Autodesk Fusion 360 part; units mm, degrees
note: some values were not read from the file. Set by a fixed rule: which sketch regions a step uses.
(part 9 of 15)
  line L7029 (253.402, -123.809) -> (253.455, -123.987)
  line L7030 (75.174, -122.125) -> (75.3489, -121.903)
  line L7031 (253.455, -123.987) -> (253.474, -124.171)
  line L7032 (253.45, -124.382) -> (253.391, -124.558)
  line L7033 (252.688, -125.107) -> (252.504, -125.121)
  line L7034 (82.7574, -124.342) -> (82.6989, -124.518)
  line L7035 (82.6989, -124.518) -> (82.6073, -124.679)
  line L7036 (82.34, -124.934) -> (82.1745, -125.017)
  line L7037 (252.53, -123.222) -> (252.715, -123.241)
  line L7038 (82.7806, -124.158) -> (82.7574, -124.342)
  line L7039 (82.6073, -124.679) -> (82.4861, -124.819)
  line L7040 (82.1991, -123.256) -> (82.3622, -123.344)
  line L7041 (82.1745, -125.017) -> (81.996, -125.067)
  line L7042 (81.996, -125.067) -> (81.8111, -125.081)
  line L7043 (82.7093, -123.769) -> (82.7629, -123.947)
  line L7044 (251.981, -124.952) -> (251.84, -124.831)
  line L7045 (251.859, -123.493) -> (252.003, -123.377)
  line L7046 (277.272, -120.321) -> (277.535, -120.423)
  line L7047 (278.68, -122.358) -> (278.642, -122.638)
  line L7048 (82.5051, -123.462) -> (82.6223, -123.606)
  line L7049 (251.74, -123.635) -> (251.859, -123.493)
  line L7050 (276.997, -120.257) -> (277.272, -120.321)
  line L7051 (82.4861, -124.819) -> (82.34, -124.934)
  line L7052 (252.32, -125.099) -> (252.143, -125.042)
  line L7053 (81.8376, -123.181) -> (82.022, -123.201)
  line L7054 (75.5533, -121.708) -> (75.7832, -121.544)
  line L7055 (253.055, -123.384) -> (253.198, -123.502)
  line L7056 (278.566, -122.91) -> (278.451, -123.168)
  line L7057 (278.604, -121.675) -> (278.664, -121.951)
  line L7058 (252.143, -125.042) -> (251.981, -124.952)
  line L7059 (251.64, -124.521) -> (251.589, -124.343)
  line L7060 (81.653, -123.198) -> (81.8376, -123.181)
  line L7061 (81.627, -125.059) -> (81.4507, -125.002)
  line L7062 (81.0324, -124.646) -> (80.9477, -124.481)
  line L7063 (278.007, -120.732) -> (278.205, -120.934)
  line L7064 (251.84, -124.831) -> (251.725, -124.686)
  line L7065 (82.7629, -123.947) -> (82.781, -124.131)
  line L7066 (252.346, -123.238) -> (252.53, -123.222)
  line L7067 (251.589, -124.343) -> (251.574, -124.158)
  line L7068 (278.373, -121.161) -> (278.507, -121.41)
  line L7069 (82.6223, -123.606) -> (82.7093, -123.769)
  line L7070 (251.594, -123.974) -> (251.65, -123.797)
  line L7071 (278.684, -122.233) -> (278.68, -122.358)
  line L7072 (278.642, -122.638) -> (278.566, -122.91)
  line L7073 (252.168, -123.291) -> (252.346, -123.238)
  line L7074 (253.198, -123.502) -> (253.315, -123.646)
  line L7075 (278.451, -123.168) -> (278.302, -123.408)
  line L7076 (82.3622, -123.344) -> (82.5051, -123.462)
  line L7077 (278.205, -120.934) -> (278.373, -121.161)
  line L7078 (80.9477, -124.481) -> (80.8966, -124.303)
  line L7079 (252.003, -123.377) -> (252.168, -123.291)
  line L7080 (76.8596, -121.25) -> (77.141, -121.274)
  line L7081 (278.507, -121.41) -> (278.604, -121.675)
  line L7082 (81.3108, -123.336) -> (81.4751, -123.251)
  line L7083 (277.782, -120.561) -> (278.007, -120.732)
  line L7084 (253.3, -124.719) -> (253.179, -124.859)
  line L7085 (253.315, -123.646) -> (253.402, -123.809)
  line L7086 (81.4751, -123.251) -> (81.653, -123.198)
  line L7087 (81.0471, -123.595) -> (81.1663, -123.453)
  line L7088 (80.9578, -123.757) -> (81.0471, -123.595)
  line L7089 (82.781, -124.131) -> (82.7806, -124.158)
  line L7090 (278.664, -121.951) -> (278.684, -122.233)
  line L7091 (277.535, -120.423) -> (277.782, -120.561)
  line L7092 (82.022, -123.201) -> (82.1991, -123.256)
  line L7093 (251.725, -124.686) -> (251.64, -124.521)
  line L7094 (251.65, -123.797) -> (251.74, -123.635)
  line L7095 (76.3004, -121.32) -> (76.5775, -121.265)
  line L7096 (251.574, -124.158) -> (251.594, -123.974)
  line L7097 (253.179, -124.859) -> (253.033, -124.974)
  line L7098 (57.8588, -124.184) -> (57.5764, -124.19)
  line L7099 (58.1375, -124.137) -> (57.8588, -124.184)
  line L7100 (55.7334, -122.69) -> (55.6827, -122.412)
  line L7101 (58.5222, -120.383) -> (58.7687, -120.521)
  line L7102 (81.1663, -123.453) -> (81.3108, -123.336)
  line L7103 (275.03, -121.108) -> (275.205, -120.887)
  line L7104 (278.12, -123.624) -> (277.91, -123.813)
  line L7105 (277.42, -124.092) -> (277.151, -124.177)
  line L7106 (59.1069, -123.584) -> (58.8964, -123.773)
  line L7107 (275.205, -120.887) -> (275.409, -120.692)
  line L7108 (276.036, -124.125) -> (275.776, -124.015)
  line L7109 (55.8229, -122.958) -> (55.7334, -122.69)
  line L7110 (275.639, -120.527) -> (275.89, -120.397)
  line L7111 (59.5912, -121.635) -> (59.6507, -121.911)
  line L7112 (57.0228, -124.085) -> (56.7626, -123.975)
  line L7113 (58.9932, -120.692) -> (59.1914, -120.894)
  line L7114 (59.5524, -122.87) -> (59.4381, -123.128)
  line L7115 (276.156, -120.304) -> (276.433, -120.248)
  line L7116 (274.836, -122.998) -> (274.747, -122.73)
  line L7117 (58.2587, -120.281) -> (58.5222, -120.383)
  line L7118 (276.433, -120.248) -> (276.715, -120.233)
  line L7119 (276.59, -124.23) -> (276.309, -124.197)
  line L7120 (274.782, -121.615) -> (274.888, -121.353)
  line L7121 (57.9835, -120.217) -> (58.2587, -120.281)
  line L7122 (274.685, -122.17) -> (274.714, -121.889)
  line L7123 (276.309, -124.197) -> (276.036, -124.125)
  line L7124 (278.302, -123.408) -> (278.12, -123.624)
  line L7125 (57.5764, -124.19) -> (57.2959, -124.157)
  line L7126 (81.2888, -124.912) -> (81.1476, -124.791)
  line L7127 (80.9017, -123.934) -> (80.9578, -123.757)
  line L7128 (274.888, -121.353) -> (275.03, -121.108)
  line L7129 (56.5206, -123.829) -> (56.3015, -123.65)
  line L7130 (56.3015, -123.65) -> (56.1098, -123.443)
  line L7131 (59.3593, -121.121) -> (59.4934, -121.37)
  line L7132 (58.7687, -120.521) -> (58.9932, -120.692)
  line L7133 (55.6716, -122.13) -> (55.7004, -121.849)
  line L7134 (276.872, -124.224) -> (276.59, -124.23)
  line L7135 (275.89, -120.397) -> (276.156, -120.304)
  line L7136 (81.4507, -125.002) -> (81.2888, -124.912)
  line L7137 (81.1476, -124.791) -> (81.0324, -124.646)
  line L7138 (277.91, -123.813) -> (277.675, -123.97)
  line L7139 (56.7626, -123.975) -> (56.5206, -123.829)
  line L7140 (59.4381, -123.128) -> (59.2886, -123.368)
  line L7141 (59.6291, -122.598) -> (59.5524, -122.87)
  line L7142 (275.534, -123.869) -> (275.315, -123.691)
  line L7143 (274.747, -122.73) -> (274.696, -122.452)
  line L7144 (274.696, -122.452) -> (274.685, -122.17)
  line L7145 (277.675, -123.97) -> (277.42, -124.092)
  line L7146 (275.123, -123.483) -> (274.962, -123.251)
  line L7147 (275.409, -120.692) -> (275.639, -120.527)
  line L7148 (276.715, -120.233) -> (276.997, -120.257)
  line L7149 (274.714, -121.889) -> (274.782, -121.615)
  line L7150 (275.776, -124.015) -> (275.534, -123.869)
  line L7151 (274.962, -123.251) -> (274.836, -122.998)
  line L7152 (59.4934, -121.37) -> (59.5912, -121.635)
  line L7153 (59.6667, -122.318) -> (59.6291, -122.598)
  line L7154 (56.1098, -123.443) -> (55.9491, -123.211)
  line L7155 (55.9491, -123.211) -> (55.8229, -122.958)
  line L7156 (81.8111, -125.081) -> (81.627, -125.059)
  line L7157 (80.8966, -124.303) -> (80.8811, -124.118)
  line L7158 (55.6827, -122.412) -> (55.6716, -122.13)
  line L7159 (275.315, -123.691) -> (275.123, -123.483)
  line L7160 (80.8811, -124.118) -> (80.9017, -123.934)
  line L7161 (277.151, -124.177) -> (276.872, -124.224)
  line L7162 (270.798, -123.464) -> (270.747, -123.286)
  line L7163 (271.016, -122.436) -> (271.161, -122.32)
  line L7164 (272.336, -123.803) -> (272.19, -123.917)
  line L7165 (59.6706, -122.193) -> (59.6667, -122.318)
  line L7166 (63.4497, -123.622) -> (63.3286, -123.763)
  line L7167 (55.8746, -121.313) -> (56.0165, -121.068)
  line L7168 (58.8964, -123.773) -> (58.6615, -123.93)
  line L7169 (56.3958, -120.652) -> (56.6256, -120.487)
  line L7170 (270.883, -123.629) -> (270.798, -123.464)
  line L7171 (62.8384, -124.01) -> (62.6535, -124.024)
  line L7172 (271.139, -123.895) -> (270.998, -123.775)
  line L7173 (63.5518, -122.713) -> (63.6053, -122.89)
  line L7174 (270.897, -122.578) -> (271.016, -122.436)
  line L7175 (270.808, -122.741) -> (270.897, -122.578)
  line L7176 (63.1825, -123.877) -> (63.017, -123.96)
  line L7177 (63.6234, -123.075) -> (63.6231, -123.101)
  line L7178 (62.6535, -124.024) -> (62.4694, -124.003)
  line L7179 (63.5413, -123.461) -> (63.4497, -123.622)
  line L7180 (272.472, -122.589) -> (272.559, -122.753)
  line L7181 (55.7685, -121.575) -> (55.8746, -121.313)
  line L7182 (271.477, -124.043) -> (271.301, -123.985)
  line L7183 (62.2931, -123.945) -> (62.1313, -123.855)
  line L7184 (62.1313, -123.855) -> (61.9901, -123.735)
  line L7185 (58.4069, -124.052) -> (58.1375, -124.137)
  line L7186 (272.607, -123.325) -> (272.549, -123.501)
  line L7187 (63.3286, -123.763) -> (63.1825, -123.877)
  line L7188 (56.8763, -120.357) -> (57.1429, -120.263)
  line L7189 (272.025, -124) -> (271.846, -124.05)
  line L7190 (62.4694, -124.003) -> (62.2931, -123.945)
  line L7191 (272.19, -123.917) -> (272.025, -124)
  line L7192 (271.503, -122.182) -> (271.688, -122.165)
  line L7193 (271.872, -122.184) -> (272.049, -122.239)
  line L7194 (63.3475, -122.405) -> (63.4647, -122.549)
  line L7195 (57.42, -120.208) -> (57.702, -120.193)
  line L7196 (272.613, -122.93) -> (272.631, -123.115)
  line L7197 (63.5998, -123.285) -> (63.5413, -123.461)
  line L7198 (59.1914, -120.894) -> (59.3593, -121.121)
  line L7199 (57.1429, -120.263) -> (57.42, -120.208)
  line L7200 (56.1914, -120.847) -> (56.3958, -120.652)
  line L7201 (59.2886, -123.368) -> (59.1069, -123.584)
  line L7202 (56.6256, -120.487) -> (56.8763, -120.357)
  line L7203 (271.161, -122.32) -> (271.325, -122.234)
  line L7204 (272.559, -122.753) -> (272.613, -122.93)
  line L7205 (272.212, -122.327) -> (272.355, -122.445)
  line L7206 (63.4647, -122.549) -> (63.5518, -122.713)
  line L7207 (57.2959, -124.157) -> (57.0228, -124.085)
  line L7208 (56.0165, -121.068) -> (56.1914, -120.847)
  line L7209 (63.6053, -122.89) -> (63.6234, -123.075)
  line L7210 (272.049, -122.239) -> (272.212, -122.327)
  line L7211 (272.549, -123.501) -> (272.457, -123.662)
  line L7212 (272.631, -123.115) -> (272.631, -123.141)
  line L7213 (63.0416, -122.199) -> (63.2047, -122.287)
  line L7214 (272.631, -123.141) -> (272.607, -123.325)
  line L7215 (57.702, -120.193) -> (57.9835, -120.217)
  line L7216 (272.355, -122.445) -> (272.472, -122.589)
  line L7217 (272.457, -123.662) -> (272.336, -123.803)
  line L7218 (55.7004, -121.849) -> (55.7685, -121.575)
  line L7219 (271.846, -124.05) -> (271.661, -124.065)
  line L7220 (271.301, -123.985) -> (271.139, -123.895)
  line L7221 (271.325, -122.234) -> (271.503, -122.182)
  line L7222 (271.661, -124.065) -> (271.477, -124.043)
  line L7223 (59.6507, -121.911) -> (59.6706, -122.193)
  line L7224 (58.6615, -123.93) -> (58.4069, -124.052)
  line L7225 (270.998, -123.775) -> (270.883, -123.629)
  line L7226 (61.9901, -123.735) -> (61.8749, -123.589)
  line L7227 (297.548, -122.852) -> (297.366, -123.068)
  line L7228 (62.3176, -122.194) -> (62.4954, -122.142)
  line L7229 (294.082, -122.442) -> (293.992, -122.174)
  line L7230 (294.369, -122.927) -> (294.208, -122.694)
  line L7231 (271.688, -122.165) -> (271.872, -122.184)
  line L7232 (297.252, -120.176) -> (297.45, -120.377)
  line L7233 (294.208, -122.694) -> (294.082, -122.442)
  line L7234 (293.959, -121.332) -> (294.028, -121.058)
  line L7235 (295.679, -119.692) -> (295.961, -119.676)
  line L7236 (270.731, -123.101) -> (270.752, -122.917)
  line L7237 (296.118, -123.667) -> (295.835, -123.674)
  line L7238 (294.275, -120.552) -> (294.45, -120.33)
  line L7239 (39.7475, -120.136) -> (39.9457, -120.337)
  line L7240 (295.835, -123.674) -> (295.555, -123.641)
  line L7241 (294.655, -120.135) -> (294.885, -119.971)
  line L7242 (293.992, -122.174) -> (293.942, -121.896)
  line L7243 (296.243, -119.701) -> (296.518, -119.765)
  line L7244 (297.926, -121.802) -> (297.888, -122.082)
  line L7245 (297.91, -121.394) -> (297.93, -121.676)
  line L7246 (297.366, -123.068) -> (297.155, -123.256)
  line L7247 (295.961, -119.676) -> (296.243, -119.701)
  line L7248 (294.45, -120.33) -> (294.655, -120.135)
  line L7249 (295.135, -119.841) -> (295.402, -119.747)
  line L7250 (297.618, -120.605) -> (297.752, -120.853)
  line L7251 (294.78, -123.312) -> (294.561, -123.134)
  line L7252 (63.2047, -122.287) -> (63.3475, -122.405)
  line L7253 (296.518, -119.765) -> (296.781, -119.867)
  line L7254 (39.5229, -119.964) -> (39.7475, -120.136)
  line L7255 (62.6801, -122.125) -> (62.8645, -122.144)
  line L7256 (294.134, -120.796) -> (294.275, -120.552)
  line L7257 (297.811, -122.354) -> (297.697, -122.612)
  line L7258 (294.885, -119.971) -> (295.135, -119.841)
  line L7259 (297.93, -121.676) -> (297.926, -121.802)
  line L7260 (63.6231, -123.101) -> (63.5998, -123.285)
  line L7261 (295.402, -119.747) -> (295.679, -119.692)
  line L7262 (63.017, -123.96) -> (62.8384, -124.01)
  line L7263 (296.921, -123.413) -> (296.666, -123.536)
  line L7264 (297.888, -122.082) -> (297.811, -122.354)
  line L7265 (297.85, -121.118) -> (297.91, -121.394)
  line L7266 (297.155, -123.256) -> (296.921, -123.413)
  line L7267 (38.7377, -119.661) -> (39.0129, -119.725)
  line L7268 (270.752, -122.917) -> (270.808, -122.741)
  line L7269 (297.752, -120.853) -> (297.85, -121.118)
  line L7270 (294.561, -123.134) -> (294.369, -122.927)
  line L7271 (297.45, -120.377) -> (297.618, -120.605)
  line L7272 (39.0129, -119.725) -> (39.2764, -119.826)
  line L7273 (39.9457, -120.337) -> (40.1135, -120.564)
  line L7274 (61.7235, -123.061) -> (61.7442, -122.877)
  line L7275 (61.739, -123.246) -> (61.7235, -123.061)
  line L7276 (62.1533, -122.28) -> (62.3176, -122.194)
  line L7277 (296.666, -123.536) -> (296.397, -123.621)
  line L7278 (61.8003, -122.7) -> (61.8896, -122.538)
  line L7279 (297.697, -122.612) -> (297.548, -122.852)
  line L7280 (296.781, -119.867) -> (297.028, -120.005)
  line L7281 (61.7442, -122.877) -> (61.8003, -122.7)
  line L7282 (61.8896, -122.538) -> (62.0088, -122.396)
  line L7283 (62.4954, -122.142) -> (62.6801, -122.125)
  line L7284 (61.7902, -123.424) -> (61.739, -123.246)
  line L7285 (61.8749, -123.589) -> (61.7902, -123.424)
  line L7286 (297.028, -120.005) -> (297.252, -120.176)
  line L7287 (270.747, -123.286) -> (270.731, -123.101)
  line L7288 (62.8645, -122.144) -> (63.0416, -122.199)
  line L7289 (62.0088, -122.396) -> (62.1533, -122.28)
  line L7290 (40.3454, -121.078) -> (40.4049, -121.354)
  line L7291 (295.022, -123.458) -> (294.78, -123.312)
  line L7292 (40.4049, -121.354) -> (40.4249, -121.636)
  line L7293 (293.931, -121.613) -> (293.959, -121.332)
  line L7294 (293.942, -121.896) -> (293.931, -121.613)
  line L7295 (40.4249, -121.636) -> (40.4209, -121.762)
  line L7296 (36.864, -122.887) -> (36.7034, -122.654)
  line L7297 (36.7034, -122.654) -> (36.5771, -122.401)
  line L7298 (295.555, -123.641) -> (295.282, -123.568)
  line L7299 (39.2764, -119.826) -> (39.5229, -119.964)
  line L7300 (296.397, -123.621) -> (296.118, -123.667)
  line L7301 (295.282, -123.568) -> (295.022, -123.458)
  line L7302 (294.028, -121.058) -> (294.134, -120.796)
  line L7303 (37.5169, -123.418) -> (37.2748, -123.272)
  line L7304 (40.1924, -122.572) -> (40.0429, -122.812)
  line L7305 (37.777, -123.528) -> (37.5169, -123.418)
  line L7306 (-49.5459, -108.174) -> (-49.4566, -108.012)
  line L7307 (-60.9097, -104.824) -> (-60.7419, -105.051)
  line L7308 (-64.152, -107.141) -> (-64.2783, -106.888)
  line L7309 (-62.6812, -104.138) -> (-62.3991, -104.123)
  line L7310 (-61.8424, -104.211) -> (-61.579, -104.313)
  line L7311 (-61.6943, -107.982) -> (-61.9636, -108.067)
  line L7312 (-64.4184, -106.342) -> (-64.4295, -106.06)
  line L7313 (-60.6077, -105.3) -> (-60.5099, -105.565)
  line L7314 (-64.3677, -106.62) -> (-64.4184, -106.342)
  line L7315 (-64.4007, -105.779) -> (-64.3326, -105.505)
  line L7316 (-64.3326, -105.505) -> (-64.2266, -105.243)
  line L7317 (-63.3385, -107.905) -> (-63.5805, -107.759)
  line L7318 (-64.0847, -104.999) -> (-63.9098, -104.777)
  line L7319 (-63.9098, -104.777) -> (-63.7054, -104.582)
  line L7320 (-62.3991, -104.123) -> (-62.1176, -104.147)
  line L7321 (-62.2423, -108.114) -> (-62.5247, -108.12)
  line L7322 (-63.5805, -107.759) -> (-63.7996, -107.581)
  line L7323 (-57.2367, -106.074) -> (-57.0596, -106.129)
  line L7324 (-38.3236, -111.199) -> (-38.5021, -111.248)
  line L7325 (-38.687, -111.263) -> (-38.8711, -111.241)
  line L7326 (-37.7352, -110.128) -> (-37.7171, -110.313)
  line L7327 (-37.7888, -109.951) -> (-37.7352, -110.128)
  line L7328 (-39.2093, -111.093) -> (-39.3505, -110.973)
  line L7329 (-38.6605, -109.363) -> (-38.4761, -109.382)
  line L7330 (241.513, -109.894) -> (241.367, -110.008)
  line L7331 (-38.012, -111.001) -> (-38.1581, -111.115)
  line L7332 (-43.9206, -107.446) -> (-43.6385, -107.431)
  line L7333 (241.789, -109.021) -> (241.808, -109.206)
  line L7334 (-39.023, -109.432) -> (-38.8451, -109.38)
  line L7335 (-39.617, -110.3) -> (-39.5963, -110.115)
  line L7336 (-44.4642, -107.595) -> (-44.1977, -107.502)
  line L7337 (241.201, -110.092) -> (241.023, -110.141)
  line L7338 (240.838, -110.156) -> (240.654, -110.134)
  line L7339 (-38.8451, -109.38) -> (-38.6605, -109.363)
  line L7340 (-44.7149, -107.725) -> (-44.4642, -107.595)
  line L7341 (-39.4656, -110.827) -> (-39.5504, -110.663)
  line L7342 (240.477, -110.076) -> (240.315, -109.986)
  line L7343 (-39.5403, -109.939) -> (-39.451, -109.776)
  line L7344 (241.634, -109.754) -> (241.513, -109.894)
  line L7345 (241.808, -109.206) -> (241.807, -109.232)
  line L7346 (241.725, -109.592) -> (241.634, -109.754)
  line L7347 (-39.0474, -111.183) -> (-39.2093, -111.093)
  line L7348 (-39.6015, -110.484) -> (-39.617, -110.3)
  line L7349 (-37.8758, -109.787) -> (-37.7888, -109.951)
  line L7350 (-38.299, -109.437) -> (-38.1359, -109.525)
  line L7351 (-45.466, -108.551) -> (-45.3241, -108.307)
  line L7352 (-39.1873, -109.518) -> (-39.023, -109.432)
  line L7353 (-39.3505, -110.973) -> (-39.4656, -110.827)
  line L7354 (-45.3241, -108.307) -> (-45.1492, -108.085)
  line L7355 (240.654, -110.134) -> (240.477, -110.076)
  line L7356 (-45.572, -108.813) -> (-45.466, -108.551)
  line L7357 (-37.8908, -110.86) -> (-38.012, -111.001)
  line L7358 (241.807, -109.232) -> (241.784, -109.416)
  line L7359 (240.174, -109.866) -> (240.059, -109.721)
  line L7360 (241.389, -108.418) -> (241.532, -108.536)
  line L7361 (241.784, -109.416) -> (241.725, -109.592)
  line L7362 (240.315, -109.986) -> (240.174, -109.866)
  line L7363 (241.649, -108.68) -> (241.736, -108.844)
  line L7364 (-39.451, -109.776) -> (-39.3318, -109.634)
  line L7365 (-39.5504, -110.663) -> (-39.6015, -110.484)
  line L7366 (241.367, -110.008) -> (241.201, -110.092)
  line L7367 (241.023, -110.141) -> (240.838, -110.156)
  line L7368 (-39.5963, -110.115) -> (-39.5403, -109.939)
  line L7369 (241.049, -108.275) -> (241.226, -108.33)
  line L7370 (241.226, -108.33) -> (241.389, -108.418)
  line L7371 (241.736, -108.844) -> (241.789, -109.021)
  line L7372 (94.447, -109.166) -> (94.4466, -109.192)
  line L7373 (240.074, -108.669) -> (240.193, -108.527)
  line L7374 (94.0282, -108.378) -> (94.1711, -108.496)
  line L7375 (94.4466, -109.192) -> (94.4234, -109.376)
  line L7376 (240.059, -109.721) -> (239.974, -109.556)
  line L7377 (239.928, -109.008) -> (239.984, -108.832)
  line L7378 (240.193, -108.527) -> (240.337, -108.411)
  line L7379 (-39.3318, -109.634) -> (-39.1873, -109.518)
  line L7380 (94.4234, -109.376) -> (94.3648, -109.552)
  line L7381 (94.3648, -109.552) -> (94.2733, -109.713)
  line L7382 (239.908, -109.193) -> (239.928, -109.008)
  line L7383 (93.8651, -108.29) -> (94.0282, -108.378)
  line L7384 (240.502, -108.325) -> (240.68, -108.273)
  line L7385 (94.2733, -109.713) -> (94.1521, -109.854)
  line L7386 (241.532, -108.536) -> (241.649, -108.68)
  line L7387 (93.8405, -110.052) -> (93.6619, -110.101)
  line L7388 (93.293, -110.094) -> (93.1166, -110.036)
  line L7389 (94.006, -109.968) -> (93.8405, -110.052)
  line L7390 (93.6619, -110.101) -> (93.4771, -110.116)
  line L7391 (93.688, -108.235) -> (93.8651, -108.29)
  line L7392 (93.4771, -110.116) -> (93.293, -110.094)
  line L7393 (240.337, -108.411) -> (240.502, -108.325)
  line L7394 (94.2882, -108.64) -> (94.3753, -108.804)
  line L7395 (240.68, -108.273) -> (240.864, -108.256)
  line L7396 (94.3753, -108.804) -> (94.4289, -108.981)
  line L7397 (94.1521, -109.854) -> (94.006, -109.968)
  line L7398 (93.1166, -110.036) -> (92.9548, -109.946)
  line L7399 (92.9548, -109.946) -> (92.8136, -109.826)
  line L7400 (239.984, -108.832) -> (240.074, -108.669)
  line L7401 (239.923, -109.377) -> (239.908, -109.193)
  line L7402 (94.1711, -108.496) -> (94.2882, -108.64)
  line L7403 (239.974, -109.556) -> (239.923, -109.377)
  line L7404 (240.864, -108.256) -> (241.049, -108.275)
  line L7405 (-47.7228, -108.549) -> (-47.7231, -108.575)
  line L7406 (-47.9987, -107.879) -> (-47.8815, -108.023)
  line L7407 (-48.3292, -109.434) -> (-48.5078, -109.484)
  line L7408 (-47.8049, -108.935) -> (-47.8965, -109.096)
  line L7409 (94.4289, -108.981) -> (94.447, -109.166)
  line L7410 (-48.0176, -109.237) -> (-48.1637, -109.351)
  line L7411 (92.5626, -109.337) -> (92.5471, -109.153)
  line L7412 (-48.3046, -107.673) -> (-48.1415, -107.761)
  line L7413 (-48.5078, -109.484) -> (-48.6926, -109.498)
  line L7414 (93.319, -108.233) -> (93.5036, -108.216)
  line L7415 (92.6984, -109.68) -> (92.6137, -109.516)
  line L7416 (-47.8815, -108.023) -> (-47.7944, -108.187)
  line L7417 (92.8136, -109.826) -> (92.6984, -109.68)
  line L7418 (92.6137, -109.516) -> (92.5626, -109.337)
  line L7419 (-47.7408, -108.364) -> (-47.7228, -108.549)
  line L7420 (-47.7464, -108.759) -> (-47.8049, -108.935)
  line L7421 (-48.6926, -109.498) -> (-48.8768, -109.476)
  line L7422 (-48.4817, -107.618) -> (-48.3046, -107.673)
  line L7423 (-47.8965, -109.096) -> (-48.0176, -109.237)
  line L7424 (93.1411, -108.285) -> (93.319, -108.233)
  line L7425 (-47.7231, -108.575) -> (-47.7464, -108.759)
  line L7426 (92.6238, -108.792) -> (92.7131, -108.629)
  line L7427 (-49.0531, -109.419) -> (-49.2149, -109.329)
  line L7428 (92.5471, -109.153) -> (92.5677, -108.968)
  line L7429 (-61.3325, -104.451) -> (-61.1079, -104.622)
  line L7430 (-49.3561, -109.208) -> (-49.4713, -109.063)
  line L7431 (-49.4713, -109.063) -> (-49.556, -108.898)
  line L7432 (-48.1415, -107.761) -> (-47.9987, -107.879)
  line L7433 (-60.5099, -105.565) -> (-60.4505, -105.841)
  line L7434 (-49.556, -108.898) -> (-49.6071, -108.72)
  line L7435 (-48.8768, -109.476) -> (-49.0531, -109.419)
  line L7436 (-60.663, -107.059) -> (-60.8125, -107.298)
  line L7437 (92.5677, -108.968) -> (92.6238, -108.792)
  line L7438 (92.9768, -108.371) -> (93.1411, -108.285)
  line L7439 (-60.4345, -106.248) -> (-60.4721, -106.528)
  line L7440 (93.5036, -108.216) -> (93.688, -108.235)
  line L7441 (-60.4305, -106.123) -> (-60.4345, -106.248)
  line L7442 (-62.1176, -104.147) -> (-61.8424, -104.211)
  line L7443 (92.7131, -108.629) -> (92.8323, -108.487)
  line L7444 (-60.4505, -105.841) -> (-60.4305, -106.123)
  line L7445 (-48.1637, -109.351) -> (-48.3292, -109.434)
  line L7446 (-47.7944, -108.187) -> (-47.7408, -108.364)
  line L7447 (92.8323, -108.487) -> (92.9768, -108.371)
  line L7448 (-48.6661, -107.599) -> (-48.4817, -107.618)
  line L7449 (-60.8125, -107.298) -> (-60.9943, -107.515)
  line L7450 (-49.3374, -107.87) -> (-49.1929, -107.754)
  line L7451 (-61.579, -104.313) -> (-61.3325, -104.451)
  line L7452 (-49.6071, -108.72) -> (-49.6227, -108.535)
  line L7453 (-49.1929, -107.754) -> (-49.0286, -107.668)
  line L7454 (-60.4721, -106.528) -> (-60.5488, -106.8)
  line L7455 (-49.6227, -108.535) -> (-49.602, -108.351)
  line L7456 (-60.9943, -107.515) -> (-61.2047, -107.703)
  line L7457 (-60.5488, -106.8) -> (-60.663, -107.059)
  line L7458 (-48.8508, -107.615) -> (-48.6661, -107.599)
  line L7459 (-49.602, -108.351) -> (-49.5459, -108.174)
  line L7460 (-61.2047, -107.703) -> (-61.4396, -107.86)
  line L7461 (-60.7419, -105.051) -> (-60.6077, -105.3)
  line L7462 (-61.1079, -104.622) -> (-60.9097, -104.824)
  line L7463 (-49.0286, -107.668) -> (-48.8508, -107.615)
  line L7464 (-49.4566, -108.012) -> (-49.3374, -107.87)
  line L7465 (-49.2149, -109.329) -> (-49.3561, -109.208)
  line L7466 (320.643, -117.486) -> (320.643, -117.513)
  line L7467 (129.692, -117.836) -> (129.748, -117.659)
  line L7468 (319.028, -116.807) -> (319.173, -116.691)
  line L7469 (15.6111, -117.473) -> (15.5878, -117.656)
  line L7470 (15.5934, -117.261) -> (15.6114, -117.446)
  line L7471 (15.5293, -117.832) -> (15.4377, -117.994)
  line L7472 (129.837, -117.496) -> (129.957, -117.354)
  line L7473 (15.4377, -117.994) -> (15.3166, -118.134)
  line L7474 (318.82, -117.112) -> (318.909, -116.949)
  line L7475 (15.3355, -116.777) -> (15.4527, -116.92)
  line L7476 (129.748, -117.659) -> (129.837, -117.496)
  line L7477 (320.202, -118.288) -> (320.037, -118.372)
  line L7478 (15.4527, -116.92) -> (15.5398, -117.084)
  line L7479 (320.484, -116.96) -> (320.571, -117.124)
  line L7480 (319.151, -118.266) -> (319.01, -118.146)
  line L7481 (130.101, -117.238) -> (130.265, -117.152)
  line L7482 (320.061, -116.61) -> (320.224, -116.698)
  line L7483 (319.173, -116.691) -> (319.337, -116.605)
  line L7484 (319.489, -118.414) -> (319.313, -118.357)
  line L7485 (15.3166, -118.134) -> (15.1705, -118.248)
  line L7486 (15.1705, -118.248) -> (15.005, -118.332)
  line L7487 (130.628, -117.083) -> (130.812, -117.102)
  line L7488 (319.858, -118.422) -> (319.673, -118.436)
  line L7489 (130.241, -118.904) -> (130.079, -118.813)
  line L7490 (318.759, -117.658) -> (318.743, -117.473)
  line L7491 (15.6114, -117.446) -> (15.6111, -117.473)
  line L7492 (320.367, -116.817) -> (320.484, -116.96)
  line L7493 (129.823, -118.548) -> (129.738, -118.383)
  line L7494 (129.957, -117.354) -> (130.101, -117.238)
  line L7495 (319.313, -118.357) -> (319.151, -118.266)
  line L7496 (319.673, -118.436) -> (319.489, -118.414)
  line L7497 (130.443, -117.1) -> (130.628, -117.083)
  line L7498 (319.884, -116.555) -> (320.061, -116.61)
  line L7499 (318.764, -117.289) -> (318.82, -117.112)
  line L7500 (15.5878, -117.656) -> (15.5293, -117.832)
  line L7501 (319.01, -118.146) -> (318.895, -118.001)
  line L7502 (318.909, -116.949) -> (319.028, -116.807)
  line L7503 (15.5398, -117.084) -> (15.5934, -117.261)
  line L7504 (318.895, -118.001) -> (318.81, -117.836)
  line L7505 (-4.8261, -114.546) -> (-4.6279, -114.748)
  line L7506 (-4.1488, -116.047) -> (-4.1527, -116.172)
  line L7507 (-5.8359, -114.071) -> (-5.5607, -114.135)
  line L7508 (-5.5607, -114.135) -> (-5.2972, -114.237)
  line L7509 (13.8776, -116.909) -> (13.9968, -116.767)
  line L7510 (-4.4601, -114.975) -> (-4.326, -115.224)
  line L7511 (-4.267, -116.724) -> (-4.3812, -116.983)
  line L7512 (14.1193, -118.226) -> (13.9781, -118.106)
  line L7513 (14.8525, -116.515) -> (15.0296, -116.57)
  line L7514 (14.6681, -116.496) -> (14.8525, -116.515)
  line L7515 (-5.0507, -114.375) -> (-4.8261, -114.546)
  line L7516 (-4.2282, -115.489) -> (-4.1687, -115.765)
  line L7517 (13.9781, -118.106) -> (13.8629, -117.961)
  line L7518 (-4.3259, -115.224) -> (-4.2282, -115.489)
  line L7519 (14.4834, -116.513) -> (14.6681, -116.496)
  line L7520 (14.8264, -118.382) -> (14.6415, -118.396)
  line L7521 (-4.1687, -115.765) -> (-4.1488, -116.047)
  line L7522 (-4.1903, -116.452) -> (-4.267, -116.724)
  line L7523 (-4.6279, -114.748) -> (-4.4601, -114.975)
  line L7524 (318.743, -117.473) -> (318.764, -117.289)
  line L7525 (319.337, -116.605) -> (319.515, -116.553)
  line L7526 (13.7883, -117.072) -> (13.8776, -116.909)
  line L7527 (15.0296, -116.57) -> (15.1927, -116.658)
  line L7528 (13.8629, -117.961) -> (13.7782, -117.796)
  line L7529 (-4.1527, -116.172) -> (-4.1903, -116.452)
  line L7530 (15.005, -118.332) -> (14.8264, -118.382)
  line L7531 (319.7, -116.536) -> (319.884, -116.555)
  line L7532 (15.1927, -116.658) -> (15.3355, -116.777)
  line L7533 (318.81, -117.836) -> (318.759, -117.658)
  line L7534 (319.515, -116.553) -> (319.7, -116.536)
  line L7535 (-7.8702, -117.065) -> (-7.9965, -116.812)
  line L7536 (-4.7125, -117.438) -> (-4.9229, -117.627)
  line L7537 (14.6415, -118.396) -> (14.4574, -118.374)
  line L7538 (13.7322, -117.248) -> (13.7883, -117.072)
  line L7539 (-8.0859, -116.544) -> (-8.1367, -116.266)
  line L7540 (14.3056, -116.565) -> (14.4834, -116.513)
  line L7541 (-6.3994, -114.062) -> (-6.1173, -114.047)
  line L7542 (-6.1173, -114.047) -> (-5.8359, -114.071)
  line L7543 (-6.5235, -118.011) -> (-6.7966, -117.939)
  line L7544 (-7.1937, -114.341) -> (-6.9431, -114.211)
  line L7545 (-8.1478, -115.984) -> (-8.119, -115.703)
  line L7546 (13.7782, -117.796) -> (13.7271, -117.617)
  line L7547 (-0.9549, -115.998) -> (-0.7778, -116.053)
  line L7548 (14.1413, -116.651) -> (14.3056, -116.565)
  line L7549 (-6.6765, -114.118) -> (-6.3994, -114.062)
  line L7550 (-5.4125, -117.906) -> (-5.6819, -117.991)
  line L7551 (-7.5179, -117.505) -> (-7.7096, -117.297)
  line L7552 (13.7115, -117.433) -> (13.7322, -117.248)
  line L7553 (-8.119, -115.703) -> (-8.0509, -115.429)
  line L7554 (-8.0509, -115.429) -> (-7.9448, -115.167)
  line L7555 (-7.8029, -114.923) -> (-7.628, -114.701)
  line L7556 (-7.4236, -114.506) -> (-7.1937, -114.341)
  line L7557 (-7.9448, -115.167) -> (-7.8029, -114.923)
  line L7558 (-7.628, -114.701) -> (-7.4236, -114.506)
  line L7559 (13.7271, -117.617) -> (13.7115, -117.433)
  line L7560 (14.4574, -118.374) -> (14.2811, -118.317)
  line L7561 (14.2811, -118.317) -> (14.1193, -118.226)
  line L7562 (-7.7096, -117.297) -> (-7.8702, -117.065)
  line L7563 (13.9968, -116.767) -> (14.1413, -116.651)
  line L7564 (-5.2972, -114.237) -> (-5.0507, -114.375)
  line L7565 (-7.9965, -116.812) -> (-8.0859, -116.544)
  line L7566 (-4.9229, -117.627) -> (-5.1578, -117.784)
  line L7567 (-0.1963, -116.955) -> (-0.2195, -117.139)
  line L7568 (-2.0752, -116.731) -> (-2.0191, -116.555)
  line L7569 (-1.9298, -116.392) -> (-1.8106, -116.25)
  line L7570 (-8.1367, -116.266) -> (-8.1478, -115.984)
  line L7571 (-7.2988, -117.683) -> (-7.5179, -117.505)
  line L7572 (-0.2195, -117.139) -> (-0.2781, -117.315)
  line L7573 (-5.6819, -117.991) -> (-5.9605, -118.038)
  line L7574 (-0.7778, -116.053) -> (-0.6147, -116.141)
  line L7575 (-1.9445, -117.443) -> (-2.0292, -117.279)
  line L7576 (-0.4908, -117.617) -> (-0.6369, -117.731)
  line L7577 (-0.2781, -117.315) -> (-0.3696, -117.476)
  line L7578 (-4.5307, -117.222) -> (-4.7125, -117.438)
  line L7579 (-1.8106, -116.25) -> (-1.6661, -116.134)
  line L7580 (-4.3812, -116.983) -> (-4.5307, -117.222)
  line L7581 (-0.4718, -116.259) -> (-0.3547, -116.403)
  line L7582 (-0.214, -116.744) -> (-0.1959, -116.929)
  line L7583 (-5.9605, -118.038) -> (-6.243, -118.044)
  line L7584 (-6.7966, -117.939) -> (-7.0567, -117.829)
  line L7585 (-0.2676, -116.567) -> (-0.214, -116.744)
  line L7586 (-1.1658, -117.879) -> (-1.3499, -117.857)
  line L7587 (-1.3239, -115.996) -> (-1.1393, -115.979)
  line L7588 (-6.9431, -114.211) -> (-6.6765, -114.118)
  line L7589 (-2.0292, -117.279) -> (-2.0803, -117.1)
  line L7590 (-2.0191, -116.555) -> (-1.9298, -116.392)
  line L7591 (-1.5018, -116.048) -> (-1.3239, -115.996)
  line L7592 (-6.243, -118.044) -> (-6.5235, -118.011)
  line L7593 (-7.0567, -117.829) -> (-7.2988, -117.683)
  line L7594 (-5.1578, -117.784) -> (-5.4125, -117.906)
  line L7595 (-2.0958, -116.916) -> (-2.0752, -116.731)
  line L7596 (-0.6147, -116.141) -> (-0.4718, -116.259)
  line L7597 (-1.6661, -116.134) -> (-1.5018, -116.048)
  line L7598 (-1.8293, -117.589) -> (-1.9445, -117.443)
  line L7599 (-0.3547, -116.403) -> (-0.2676, -116.567)
  line L7600 (-1.6881, -117.709) -> (-1.8293, -117.589)
  line L7601 (215.93, -116.898) -> (215.77, -116.665)
  line L7602 (218.814, -114.147) -> (219.012, -114.348)
  line L7603 (218.079, -113.736) -> (218.343, -113.838)
  line L7604 (218.927, -117.039) -> (218.717, -117.228)
  line L7605 (216.341, -117.284) -> (216.122, -117.105)
  line L7606 (-1.1393, -115.979) -> (-0.9549, -115.998)
  line L7607 (-0.6369, -117.731) -> (-0.8024, -117.815)
  line L7608 (-0.8024, -117.815) -> (-0.981, -117.864)
  line L7609 (215.554, -116.145) -> (215.503, -115.867)
  line L7610 (219.491, -115.647) -> (219.487, -115.773)
  line L7611 (218.589, -113.976) -> (218.814, -114.147)
  line L7612 (219.109, -116.823) -> (218.927, -117.039)
  line L7613 (-0.1959, -116.929) -> (-0.1963, -116.955)
  line L7614 (216.843, -117.539) -> (216.583, -117.429)
  line L7615 (219.412, -115.089) -> (219.471, -115.365)
  line L7616 (217.679, -117.638) -> (217.397, -117.645)
  line L7617 (216.583, -117.429) -> (216.341, -117.284)
  line L7618 (217.116, -117.612) -> (216.843, -117.539)
  line L7619 (217.397, -117.645) -> (217.116, -117.612)
  line L7620 (215.77, -116.665) -> (215.643, -116.413)
  line L7621 (217.958, -117.592) -> (217.679, -117.638)
  line L7622 (217.804, -113.672) -> (218.079, -113.736)
  line L7623 (-2.0803, -117.1) -> (-2.0958, -116.916)
  line L7624 (218.343, -113.838) -> (218.589, -113.976)
  line L7625 (219.012, -114.348) -> (219.18, -114.576)
  line L7626 (216.122, -117.105) -> (215.93, -116.898)
  line L7627 (219.471, -115.365) -> (219.491, -115.647)
  line L7628 (215.643, -116.413) -> (215.554, -116.145)
  line L7629 (-0.981, -117.864) -> (-1.1658, -117.879)
  line L7630 (-1.5263, -117.799) -> (-1.6881, -117.709)
  line L7631 (-1.3499, -117.857) -> (-1.5263, -117.799)
  line L7632 (-0.3696, -117.476) -> (-0.4908, -117.617)
  line L7633 (219.487, -115.773) -> (219.45, -116.053)
  line L7634 (219.314, -114.824) -> (219.412, -115.089)
  line L7635 (219.373, -116.325) -> (219.259, -116.583)
  line L7636 (219.45, -116.053) -> (219.373, -116.325)
  line L7637 (219.259, -116.583) -> (219.109, -116.823)
  line L7638 (219.18, -114.576) -> (219.314, -114.824)
  line L7639 (218.717, -117.228) -> (218.482, -117.385)
  line L7640 (218.482, -117.385) -> (218.227, -117.507)
  line L7641 (216.216, -114.106) -> (216.446, -113.942)
  line L7642 (117.451, -113.696) -> (117.715, -113.798)
  line L7643 (118.384, -114.308) -> (118.552, -114.536)
  line L7644 (216.012, -114.301) -> (216.216, -114.106)
  line L7645 (118.186, -114.107) -> (118.384, -114.308)
  line L7646 (117.961, -113.936) -> (118.186, -114.107)
  line L7647 (118.822, -116.013) -> (118.745, -116.285)
  line L7648 (118.481, -116.783) -> (118.3, -116.999)
  line L7649 (117.715, -113.798) -> (117.961, -113.936)
  line L7650 (118.631, -116.543) -> (118.481, -116.783)
  line L7651 (218.227, -117.507) -> (217.958, -117.592)
  line L7652 (217.523, -113.648) -> (217.804, -113.672)
  line L7653 (117.176, -113.632) -> (117.451, -113.696)
  line L7654 (118.863, -115.607) -> (118.859, -115.733)
  line L7655 (118.859, -115.733) -> (118.822, -116.013)
  line L7656 (217.24, -113.663) -> (217.523, -113.648)
  line L7657 (118.3, -116.999) -> (118.089, -117.188)
  line L7658 (118.089, -117.188) -> (117.854, -117.344)
  line L7659 (215.589, -115.029) -> (215.695, -114.767)
  line L7660 (118.745, -116.285) -> (118.631, -116.543)
  line L7661 (215.521, -115.303) -> (215.589, -115.029)
  line L7662 (118.843, -115.325) -> (118.863, -115.607)
  line L7663 (216.697, -113.812) -> (216.963, -113.718)
  line L7664 (117.854, -117.344) -> (117.6, -117.467)
  line L7665 (216.963, -113.718) -> (217.24, -113.663)
  line L7666 (118.552, -114.536) -> (118.686, -114.784)
  line L7667 (118.784, -115.049) -> (118.843, -115.325)
  line L7668 (215.503, -115.867) -> (215.492, -115.584)
  line L7669 (118.686, -114.784) -> (118.784, -115.049)
  line L7670 (309.694, -118.3) -> (309.878, -118.32)
  line L7671 (24.8581, -118.28) -> (25.0352, -118.334)
  line L7672 (203.924, -117.143) -> (204.101, -117.197)
  line L7673 (204.601, -118.46) -> (204.51, -118.621)
  line L7674 (23.8832, -118.674) -> (24.0024, -118.531)
  line L7675 (204.683, -118.1) -> (204.66, -118.284)
  line L7676 (308.758, -119.053) -> (308.814, -118.876)
  line L7677 (204.101, -117.197) -> (204.265, -117.286)
  line L7678 (24.4891, -118.277) -> (24.6737, -118.26)
  line L7679 (308.738, -119.237) -> (308.758, -119.053)
  line L7680 (23.7939, -118.836) -> (23.8832, -118.674)
  line L7681 (204.51, -118.621) -> (204.388, -118.761)
  line L7682 (24.3112, -118.329) -> (24.4891, -118.277)
  line L7683 (204.242, -118.875) -> (204.077, -118.959)
  line L7684 (204.077, -118.959) -> (203.898, -119.009)
  line L7685 (23.8686, -119.725) -> (23.7838, -119.56)
  line L7686 (204.265, -117.286) -> (204.407, -117.404)
  line L7687 (23.7172, -119.197) -> (23.7378, -119.013)
  line L7688 (204.525, -117.547) -> (204.612, -117.711)
  line L7689 (130.812, -117.102) -> (130.989, -117.157)
  line L7690 (203.898, -119.009) -> (203.713, -119.023)
  line L7691 (203.529, -119.001) -> (203.353, -118.944)
  line L7692 (24.1249, -119.99) -> (23.9837, -119.87)
  line L7693 (24.0024, -118.531) -> (24.1469, -118.415)
  line L7694 (23.7838, -119.56) -> (23.7327, -119.382)
  line L7695 (23.7327, -119.382) -> (23.7172, -119.197)
  line L7696 (204.665, -117.889) -> (204.683, -118.073)
  line L7697 (204.66, -118.284) -> (204.601, -118.46)
  line L7698 (23.7378, -119.013) -> (23.7939, -118.836)
  line L7699 (202.783, -118.06) -> (202.804, -117.876)
  line L7700 (204.683, -118.073) -> (204.683, -118.1)
  line L7701 (24.1469, -118.415) -> (24.3112, -118.329)
  line L7702 (204.407, -117.404) -> (204.525, -117.547)
  line L7703 (204.388, -118.761) -> (204.242, -118.875)
  line L7704 (23.9837, -119.87) -> (23.8686, -119.725)
  line L7705 (204.612, -117.711) -> (204.665, -117.889)
  line L7706 (203.713, -119.023) -> (203.529, -119.001)
  line L7707 (24.6737, -118.26) -> (24.8581, -118.28)
  line L7708 (202.804, -117.876) -> (202.86, -117.699)
  line L7709 (131.571, -118.033) -> (131.571, -118.06)
  line L7710 (131.397, -118.581) -> (131.276, -118.721)
  line L7711 (203.069, -117.394) -> (203.213, -117.278)
  line L7712 (203.377, -117.192) -> (203.555, -117.14)
  line L7713 (130.965, -118.919) -> (130.786, -118.969)
  line L7714 (202.86, -117.699) -> (202.949, -117.536)
  line L7715 (203.74, -117.123) -> (203.924, -117.143)
  line L7716 (130.417, -118.961) -> (130.241, -118.904)
  line L7717 (129.671, -118.02) -> (129.692, -117.836)
  line L7718 (320.224, -116.698) -> (320.367, -116.817)
  line L7719 (129.738, -118.383) -> (129.687, -118.205)
  line L7720 (130.989, -117.157) -> (131.152, -117.246)
  line L7721 (202.799, -118.245) -> (202.783, -118.06)
  line L7722 (320.469, -118.034) -> (320.348, -118.174)
  line L7723 (320.348, -118.174) -> (320.202, -118.288)
  line L7724 (320.625, -117.302) -> (320.643, -117.486)
  line L7725 (320.643, -117.513) -> (320.619, -117.697)
  line L7726 (320.037, -118.372) -> (319.858, -118.422)
  line L7727 (131.489, -118.419) -> (131.397, -118.581)
  line L7728 (130.786, -118.969) -> (130.601, -118.983)
  line L7729 (320.571, -117.124) -> (320.625, -117.302)
  line L7730 (130.601, -118.983) -> (130.417, -118.961)
  line L7731 (131.276, -118.721) -> (131.13, -118.835)
  line L7732 (131.553, -117.849) -> (131.571, -118.033)
  line L7733 (131.295, -117.364) -> (131.412, -117.507)
  line L7734 (203.05, -118.733) -> (202.935, -118.588)
  line L7735 (131.412, -117.507) -> (131.5, -117.671)
  line L7736 (131.5, -117.671) -> (131.553, -117.849)
  line L7737 (130.079, -118.813) -> (129.938, -118.693)
  line L7738 (202.85, -118.423) -> (202.799, -118.245)
  line L7739 (129.687, -118.205) -> (129.671, -118.02)
  line L7740 (129.938, -118.693) -> (129.823, -118.548)
  line L7741 (130.265, -117.152) -> (130.443, -117.1)
  line L7742 (320.619, -117.697) -> (320.561, -117.872)
  line L7743 (203.555, -117.14) -> (203.74, -117.123)
  line L7744 (202.949, -117.536) -> (203.069, -117.394)
  line L7745 (320.561, -117.872) -> (320.469, -118.034)
  line L7746 (203.213, -117.278) -> (203.377, -117.192)
  line L7747 (202.935, -118.588) -> (202.85, -118.423)
  line L7748 (131.548, -118.244) -> (131.489, -118.419)
  line L7749 (131.571, -118.06) -> (131.548, -118.244)
  line L7750 (203.191, -118.853) -> (203.05, -118.733)
  line L7751 (131.152, -117.246) -> (131.295, -117.364)
  line L7752 (131.13, -118.835) -> (130.965, -118.919)
  line L7753 (203.353, -118.944) -> (203.191, -118.853)
  line L7754 (28.419, -112.697) -> (28.5197, -112.448)
  line L7755 (-18.9746, -113.436) -> (-18.9565, -113.621)
  line L7756 (-19.5384, -112.745) -> (-19.3753, -112.833)
  line L7757 (-24.0578, -110.929) -> (-23.8113, -111.067)
  line L7758 (-24.4425, -114.683) -> (-24.7211, -114.73)
  line L7759 (-26.7571, -113.504) -> (-26.8465, -113.236)
  line L7760 (-24.7211, -114.73) -> (-25.0036, -114.736)
  line L7761 (-26.5635, -111.615) -> (-26.3886, -111.393)
  line L7762 (-18.9565, -113.621) -> (-18.9569, -113.647)
  line L7763 (-29.2381, -111.187) -> (-29.1209, -111.331)
  line L7764 (-20.5712, -112.942) -> (-20.4267, -112.826)
  line L7765 (-25.0036, -114.736) -> (-25.2841, -114.703)
  line L7766 (-19.0387, -114.007) -> (-19.1302, -114.168)
  line L7767 (-19.2324, -112.951) -> (-19.1152, -113.095)
  line L7768 (-26.8973, -112.958) -> (-26.9084, -112.676)
  line L7769 (-25.4371, -110.81) -> (-25.16, -110.754)
  line L7770 (-26.0594, -114.375) -> (-26.2784, -114.197)
  line L7771 (-26.8465, -113.236) -> (-26.8973, -112.958)
  line L7772 (-26.1842, -111.198) -> (-25.9543, -111.033)
  line L7773 (-25.2841, -114.703) -> (-25.5572, -114.631)
  line L7774 (-25.7036, -110.903) -> (-25.4371, -110.81)
  line L7775 (-25.8173, -114.521) -> (-26.0594, -114.375)
  line L7776 (-26.8115, -112.121) -> (-26.7054, -111.859)
  line L7777 (-26.7054, -111.859) -> (-26.5635, -111.615)
  line L7778 (-19.0282, -113.259) -> (-18.9746, -113.436)
  line L7779 (-25.16, -110.754) -> (-24.8779, -110.739)
  line L7780 (-26.4702, -113.989) -> (-26.6308, -113.757)
  line L7781 (-19.7155, -112.69) -> (-19.5384, -112.745)
  line L7782 (-19.1152, -113.095) -> (-19.0282, -113.259)
  line L7783 (-25.5572, -114.631) -> (-25.8173, -114.521)
  line L7784 (28.6545, -112.216) -> (28.8207, -112.005)
  line L7785 (-26.6308, -113.757) -> (-26.7571, -113.504)
  line L7786 (-24.8779, -110.739) -> (-24.5965, -110.763)
  line L7787 (-23.0865, -111.916) -> (-22.9888, -112.181)
  line L7788 (-19.3753, -112.833) -> (-19.2324, -112.951)
  line L7789 (-26.2784, -114.197) -> (-26.4702, -113.989)
  line L7790 (-26.8796, -112.395) -> (-26.8115, -112.121)
  line L7791 (-26.9084, -112.676) -> (-26.8796, -112.395)
  line L7792 (-26.3886, -111.393) -> (-26.1842, -111.198)
  line L7793 (-25.9543, -111.033) -> (-25.7036, -110.903)
  line L7794 (-30.2925, -112.727) -> (-30.4543, -112.637)
  line L7795 (-29.9321, -112.806) -> (-30.1162, -112.784)
  line L7796 (-30.1162, -112.784) -> (-30.2925, -112.727)
  line L7797 (-19.9264, -114.571) -> (-20.1105, -114.549)
  line L7798 (-29.0338, -111.495) -> (-28.9803, -111.672)
  line L7799 (-20.1105, -114.549) -> (-20.2869, -114.491)
  line L7800 (-20.6904, -113.084) -> (-20.5712, -112.942)
  line L7801 (-19.7416, -114.556) -> (-19.9264, -114.571)
  line L7802 (-20.4487, -114.401) -> (-20.5899, -114.281)
  line L7803 (-29.1209, -111.331) -> (-29.0338, -111.495)
  line L7804 (-20.8358, -113.423) -> (-20.7797, -113.247)
  line L7805 (-30.4324, -111.062) -> (-30.268, -110.976)
  line L7806 (-29.257, -112.545) -> (-29.4031, -112.659)
  line L7807 (-29.9055, -110.907) -> (-29.7211, -110.926)
  line L7808 (236.953, -108.416) -> (237.177, -108.588)
  line L7809 (237.177, -108.588) -> (237.376, -108.789)
  line L7810 (236.443, -108.176) -> (236.706, -108.278)
  line L7811 (-30.696, -111.32) -> (-30.5768, -111.178)
  line L7812 (-28.9858, -112.067) -> (-29.0443, -112.243)
  line L7813 (-28.9803, -111.672) -> (-28.9622, -111.857)
  line L7814 (-28.9622, -111.857) -> (-28.9625, -111.883)
  line L7815 (237.855, -110.088) -> (237.851, -110.214)
  line L7816 (-19.563, -114.507) -> (-19.7416, -114.556)
  line L7817 (-30.7853, -111.482) -> (-30.696, -111.32)
  line L7818 (-30.8466, -112.028) -> (-30.8621, -111.843)
  line L7819 (-29.7211, -110.926) -> (-29.544, -110.981)
  line L7820 (235.207, -111.98) -> (234.947, -111.87)
  line L7821 (-28.9625, -111.883) -> (-28.9858, -112.067)
  line L7822 (234.294, -111.339) -> (234.133, -111.106)
  line L7823 (-20.7898, -113.971) -> (-20.8409, -113.792)
  line L7824 (-30.7955, -112.206) -> (-30.8466, -112.028)
  line L7825 (-29.5686, -112.742) -> (-29.7472, -112.792)
  line L7826 (-29.0443, -112.243) -> (-29.1359, -112.404)
  line L7827 (-20.5899, -114.281) -> (-20.7051, -114.135)
  line L7828 (-18.9569, -113.647) -> (-18.9801, -113.831)
  line L7829 (-19.3975, -114.423) -> (-19.563, -114.507)
  line L7830 (-20.8409, -113.792) -> (-20.8564, -113.608)
  line L7831 (-29.544, -110.981) -> (-29.3809, -111.069)
  line L7832 (-19.8999, -112.671) -> (-19.7155, -112.69)
  line L7833 (-29.3809, -111.069) -> (-29.2381, -111.187)
  line L7834 (-30.268, -110.976) -> (-30.0902, -110.923)
  line L7835 (-19.1302, -114.168) -> (-19.2514, -114.309)
  line L7836 (-20.2624, -112.74) -> (-20.0845, -112.688)
  line L7837 (-30.5955, -112.516) -> (-30.7107, -112.371)
  line L7838 (-19.2514, -114.309) -> (-19.3975, -114.423)
  line L7839 (-20.7797, -113.247) -> (-20.6904, -113.084)
  line L7840 (-20.7051, -114.135) -> (-20.7898, -113.971)
  line L7841 (-29.7472, -112.792) -> (-29.9321, -112.806)
  line L7842 (236.706, -108.278) -> (236.953, -108.416)
  line L7843 (-29.1359, -112.404) -> (-29.257, -112.545)
  line L7844 (-29.4031, -112.659) -> (-29.5686, -112.742)
  line L7845 (-30.5768, -111.178) -> (-30.4324, -111.062)
  line L7846 (-30.0902, -110.923) -> (-29.9055, -110.907)
  line L7847 (-30.8414, -111.659) -> (-30.7853, -111.482)
  line L7848 (-30.4543, -112.637) -> (-30.5955, -112.516)
  line L7849 (-30.8621, -111.843) -> (-30.8414, -111.659)
  line L7850 (-30.7107, -112.371) -> (-30.7955, -112.206)
  line L7851 (-18.9801, -113.831) -> (-19.0387, -114.007)
  line L7852 (-20.8564, -113.608) -> (-20.8358, -113.423)
  line L7853 (236.168, -108.113) -> (236.443, -108.176)
  line L7854 (-20.2869, -114.491) -> (-20.4487, -114.401)
  line L7855 (-20.4267, -112.826) -> (-20.2624, -112.74)
  line L7856 (-20.0845, -112.688) -> (-19.8999, -112.671)
  line L7857 (234.947, -111.87) -> (234.705, -111.724)
  line L7858 (234.705, -111.724) -> (234.486, -111.546)
  line L7859 (234.007, -110.853) -> (233.918, -110.585)
  line L7860 (237.851, -110.214) -> (237.813, -110.494)
  line L7861 (236.322, -112.033) -> (236.043, -112.079)
  line L7862 (233.918, -110.585) -> (233.867, -110.307)
  line L7863 (237.473, -111.264) -> (237.291, -111.48)
  line L7864 (236.043, -112.079) -> (235.761, -112.086)
  line L7865 (237.835, -109.806) -> (237.855, -110.088)
  line L7866 (233.856, -110.025) -> (233.884, -109.744)
  line L7867 (235.48, -112.053) -> (235.207, -111.98)
  line L7868 (237.813, -110.494) -> (237.736, -110.766)
  line L7869 (236.591, -111.948) -> (236.322, -112.033)
  line L7870 (233.867, -110.307) -> (233.856, -110.025)
  line L7871 (235.06, -108.253) -> (235.327, -108.159)
  line L7872 (100.458, -110.454) -> (100.382, -110.725)
  line L7873 (234.133, -111.106) -> (234.007, -110.853)
  line L7874 (237.291, -111.48) -> (237.081, -111.668)
  line L7875 (235.886, -108.088) -> (236.168, -108.113)
  line L7876 (237.622, -111.024) -> (237.473, -111.264)
  line L7877 (237.376, -108.789) -> (237.543, -109.016)
  line L7878 (237.543, -109.016) -> (237.678, -109.265)
  line L7879 (237.081, -111.668) -> (236.846, -111.825)
  line L7880 (234.059, -109.208) -> (234.201, -108.964)
  line L7881 (237.678, -109.265) -> (237.775, -109.53)
  line L7882 (234.81, -108.383) -> (235.06, -108.253)
  line L7883 (100.496, -110.174) -> (100.458, -110.454)
  line L7884 (100.48, -109.766) -> (100.5, -110.048)
  line L7885 (100.5, -110.048) -> (100.496, -110.174)
  line L7886 (237.775, -109.53) -> (237.835, -109.806)
  line L7887 (100.118, -111.224) -> (99.936, -111.44)
  line L7888 (233.953, -109.47) -> (234.059, -109.208)
  line L7889 (99.936, -111.44) -> (99.7256, -111.628)
  line L7890 (236.846, -111.825) -> (236.591, -111.948)
  line L7891 (235.761, -112.086) -> (235.48, -112.053)
  line L7892 (237.736, -110.766) -> (237.622, -111.024)
  line L7893 (234.486, -111.546) -> (234.294, -111.339)
  line L7894 (233.884, -109.744) -> (233.953, -109.47)
  line L7895 (234.375, -108.742) -> (234.58, -108.547)
  line L7896 (100.323, -109.225) -> (100.42, -109.49)
  line L7897 (100.188, -108.976) -> (100.323, -109.225)
  line L7898 (235.327, -108.159) -> (235.604, -108.104)
  line L7899 (100.382, -110.725) -> (100.267, -110.984)
  line L7900 (99.5978, -108.376) -> (99.8224, -108.548)
  line L7901 (234.58, -108.547) -> (234.81, -108.383)
  line L7902 (100.267, -110.984) -> (100.118, -111.224)
  line L7903 (99.8224, -108.548) -> (100.021, -108.749)
  line L7904 (100.42, -109.49) -> (100.48, -109.766)
  line L7905 (100.021, -108.749) -> (100.188, -108.976)
  line L7906 (99.7256, -111.628) -> (99.4907, -111.785)
  line L7907 (235.604, -108.104) -> (235.886, -108.088)
  line L7908 (196.943, -98.8958) -> (197.111, -99.1231)
  line L7909 (195.889, -102.139) -> (195.611, -102.186)
  line L7910 (99.3513, -108.238) -> (99.5978, -108.376)
  line L7911 (195.611, -102.186) -> (195.328, -102.192)
  line L7912 (195.328, -102.192) -> (195.048, -102.159)
  line L7913 (99.0879, -108.136) -> (99.3513, -108.238)
  line L7914 (234.201, -108.964) -> (234.375, -108.742)
  line L7915 (197.111, -99.1231) -> (197.245, -99.3717)
  line L7916 (193.862, -101.445) -> (193.701, -101.213)
  line L7917 (197.403, -99.9129) -> (197.423, -100.195)